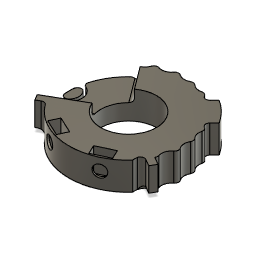
thumbwheelSmall (Autodesk Fusion 360 design; units mm, degrees)
Autodesk Fusion 360 part; units mm, degrees
note: some values were not read from the file. Chosen so that the rebuilt part matches the saved one: which face or edge a step refers to; which pieces of a blend or face edit are solid. Set by a fixed rule: which sketch regions a step uses.
sketch "Sketch1" plane through (0, 0, 0) normal (0, 1, 0) x (1, 0, 0)
  circle A0 centre (0, 0) radius 7
  circle A1 centre (0, 0) radius 15
  line L0 (0, -32.840125) -> (0, 23.247025)
  line L1 (-28.284272, 0) -> (28.284272, 0)
  line L2 (6.339274, 13.594617) -> (-6.339274, -13.594617)
  line L3 (6.339274, 13.594617) -> (-6.339274, -13.594617)
  line L4 (-6.339274, 13.594617) -> (6.339274, -13.594617)
  circle A2 centre (-15, 0) radius 2.5
  circle A3 centre (-15, 0) radius 3.25
  circle A4 centre (0, 16.5) radius 2.5
  circle A5 centre (4.270514, 15.937776) radius 2.5
  circle A6 centre (8.25, 14.289419) radius 2.5
  circle A7 centre (11.667262, 11.667262) radius 2.5
  circle A8 centre (14.289419, 8.25) radius 2.5
  circle A9 centre (15.937776, 4.270514) radius 2.5
  circle A10 centre (16.5, 0) radius 2.5
  circle A11 centre (0, 0) radius 16.5
  circle A12 centre (-4.942275, 15.742424) radius 2.5
  circle A13 centre (15.742424, -4.942275) radius 2.5
  circle A14 centre (-9.430713, 13.539263) radius 2.5
  circle A15 centre (13.539263, -9.430713) radius 2.5
  line L5 (-4.088772, -14.092354) -> (-8.167157, -12.190572)
  line L6 (-8.167157, -12.190572) -> (-7.110612, -9.924802)
  line L7 (-7.110612, -9.924802) -> (-3.032227, -11.826585)
  line L8 (-3.032227, -11.826585) -> (-4.088772, -14.092354)
  line L9 (-4.088772, -14.092354) -> (-7.110612, -9.924802) construction
  line L10 (-8.167157, -12.190572) -> (-3.032227, -11.826585) construction
  line L11 (4.088772, -14.092354) -> (8.167157, -12.190572)
  line L12 (7.110612, -9.924802) -> (3.032227, -11.826585)
  line L13 (4.088772, -14.092354) -> (7.110612, -9.924802) construction
  line L14 (3.032227, -11.826585) -> (4.088772, -14.092354)
  line L15 (8.167157, -12.190572) -> (3.032227, -11.826585) construction
  line L16 (8.167157, -12.190572) -> (7.110612, -9.924802)
  line L17 (0, 0) -> (11.667262, 11.667262)
  line L18 (12.062872, 7.113124) -> (7.113124, 12.062872)
  line L19 (7.113124, 12.062872) -> (11.271652, 16.2214)
  line L20 (11.271652, 16.2214) -> (16.2214, 11.271652)
  line L21 (16.2214, 11.271652) -> (12.062872, 7.113124)
  line L22 (12.062872, 7.113124) -> (11.271652, 16.2214) construction
  line L23 (7.113124, 12.062872) -> (16.2214, 11.271652) construction
  point P0 (-5.599692, -12.008578)
  point P1 (6.339274, -13.594617)
  point P2 (6.339274, -13.594617)
  point P3 (5.599692, -12.008578)
  point P4 (11.667262, 11.667262)
  dimension "d1" = 14
  dimension "d2" = 30
  dimension "d3" = 25
  dimension "d6" = 5
  dimension "d7" = 6.5
  dimension "d8" = 5
  dimension "d10" = -90
  dimension "d36" = 5
  dimension "d37" = 5
  dimension "d38" = 5
  dimension "d39" = 5
  dimension "d47" = 4.5
  dimension "d48" = 2.5
  dimension "d49" = 0.5
  dimension "d60" = 45
  dimension "d61" = 33
  dimension "d62" = 7
  constraint coincident A0.centre A1.centre
  constraint concentric A0 A1
  constraint coincident A0.centre L0
  constraint coincident A0.centre L1
  constraint vertical L0
  constraint horizontal L1
  constraint coincident A0.centre L2
  constraint coincident L1 A2.centre
  constraint coincident A1 A2.centre
  constraint concentric A2 A3
  constraint coincident L0 A4.centre
  constraint concentric A0 A11
  constraint coincident A10.centre A11
  constraint tangent A4 A12
  constraint tangent A12 A14
  constraint tangent A10 A13
  constraint tangent A13 A15
  constraint coincident L3 A0.centre
  constraint perpendicular L5 L6
  constraint parallel L5 L7
  constraint parallel L6 L8
  constraint perpendicular L3 L7
  constraint perpendicular L18 L19
  constraint parallel L18 L20
  constraint parallel L19 L21
  constraint perpendicular L17 L20
  measures "d1" diameter of A0
  measures "d2" diameter of A1
  measures "d3" angle of L0 L2
  measures "d6" diameter of A2
  measures "d7" diameter of A3
  measures "d8" diameter of A4
  measures "d36" diameter of A12
  measures "d37" diameter of A13
  measures "d38" diameter of A14
  measures "d39" diameter of A15
  measures "d60" angle of L1 L17
  measures "d61" diameter of A11
extrude "Extrude1" add sketch "Sketch1" along normal blind 7 contours A0 A1 L1 L4 A10 A13 A15 L11 L12 L16 | A0 A1 L1 A8 A9 A10 L17 L18 | A0 L2 L3 A6 L17 L18 | A0 A1 L0 L4 L11 L12 L14 | A0 A1 L0 L2 L3 A4 A5 A6 | A1 A6 A7 L17 L18 | A1 A7 A8 L17 L18 | A0 A1 L0 L2 L3 L5 L7 L8 | A0 A1 L0 L4 A4 A12 | A0 A1 L1 L4 A3 A14 | A0 A1 L1 L2 L3 A3 L5 L6 L7 | A1 A7 L17 | A1 A7 L17 | A1 A8 L21 | A1 A6 L19 | A1 A6 A7 A11 L17 | A1 A6 A7 | A1 A7 A8 | A1 A7 A8 A11 L17 | A1 A7 A8 A11 L21 | A1 A6 A7 A11 L19 | A1 L1 A2 | A1 L1 A2 | A6 A7 A11 | A7 A8 A11 picked at (7.909113, -7.597993) picked at (9.068114, 6.987484) picked at (7.014257, 9.04726) picked at (1.010742, -11.275528) picked at (1.56298, 11.612023) picked at (8.936312, 10.634324) picked at (10.634324, 8.936312) picked at (-1.010742, -11.275528) picked at (-1.757181, 11.566014) picked at (-10.789506, 3.925439) picked at (-8.435636, -7.427336) picked at (10.608392, 10.139282) picked at (10.139282, 10.608392) picked at (12.382065, 7.951605) picked at (7.951605, 12.382065) picked at (10.248165, 11.960008) picked at (9.148205, 11.912312) picked at (11.912312, 9.148205) picked at (11.960008, 10.248165) picked at (12.961206, 8.95232) picked at (8.95232, 12.961206) picked at (-14.195535, -0.522211) picked at (-14.195535, 0.522211) picked at (9.924324, 12.871109) picked at (12.871109, 9.924324) makes body 1 at (8.102453, 7, -7.979068) makes body 2 at (-12.801016, 2.333333, -1.189314)
sketch "Sketch2" plane through (0, 0, 0) normal (0, -1, 0) x (1, 0, 0)
  arc A0 (8.926881, -13.876628) -> (13.876628, -8.926881) centre (0, 0) ccw
  line L0 (13.876628, -8.926881) -> (12.062872, -7.113124)
  arc A1 (13.836943, -5.791288) -> (12.062872, -7.113124) centre (14.289419, -8.25) ccw
  arc A2 (13.836943, -5.791288) -> (13.879255, -5.689137) centre (0, 0) ccw
  arc A3 (14.864356, -2.01269) -> (13.879255, -5.689137) centre (15.937776, -4.270514) ccw
  arc A4 (14.864356, -2.01269) -> (14.878788, -1.903069) centre (0, 0) ccw
  arc A5 (14.878788, 1.903069) -> (14.878788, -1.903069) centre (16.5, 0) ccw
  arc A6 (14.878788, 1.903069) -> (14.765678, 2.640978) centre (0, 0) ccw
  arc A7 (13.625618, 6.272362) -> (14.765678, 2.640978) centre (15.742424, 4.942275) ccw
  arc A8 (13.625618, 6.272362) -> (13.296674, 6.942511) centre (0, 0) ccw
  arc A9 (11.121244, 10.065681) -> (13.296674, 6.942511) centre (13.539263, 9.430713) ccw
  arc A10 (11.121244, 10.065681) -> (-14.647917, 3.230873) centre (0, 0) ccw
  arc A11 (-14.647917, -3.230873) -> (-14.647917, 3.230873) centre (-15, 0) ccw
  arc A12 (-14.647917, -3.230873) -> (-10.065681, -11.121244) centre (0, 0) ccw
  arc A13 (-6.942511, -13.296674) -> (-10.065681, -11.121244) centre (-9.430713, -13.539263) ccw
  arc A14 (-6.942511, -13.296674) -> (-6.272362, -13.625618) centre (0, 0) ccw
  arc A15 (-2.640978, -14.765678) -> (-6.272362, -13.625618) centre (-4.942275, -15.742424) ccw
  arc A16 (-2.640978, -14.765678) -> (-1.903069, -14.878788) centre (0, 0) ccw
  arc A17 (1.903069, -14.878788) -> (-1.903069, -14.878788) centre (0, -16.5) ccw
  arc A18 (1.903069, -14.878788) -> (2.01269, -14.864356) centre (0, 0) ccw
  arc A19 (5.689137, -13.879255) -> (2.01269, -14.864356) centre (4.270514, -15.937776) ccw
  arc A20 (5.689137, -13.879255) -> (5.791288, -13.836943) centre (0, 0) ccw
  arc A21 (7.113124, -12.062872) -> (5.791288, -13.836943) centre (8.25, -14.289419) ccw
  line L1 (7.113124, -12.062872) -> (8.926881, -13.876628)
  circle A22 centre (0, 0) radius 7
  line L2 (-8.167157, 12.190572) -> (-4.088772, 14.092354)
  line L3 (-4.088772, 14.092354) -> (-3.032227, 11.826585)
  line L4 (-3.032227, 11.826585) -> (-7.110612, 9.924802)
  line L5 (-7.110612, 9.924802) -> (-8.167157, 12.190572)
  line L6 (7.110612, 9.924802) -> (3.032227, 11.826585)
  line L7 (3.032227, 11.826585) -> (4.088772, 14.092354)
  line L8 (4.088772, 14.092354) -> (8.167157, 12.190572)
  line L9 (8.167157, 12.190572) -> (7.110612, 9.924802)
  arc A23 (-14.791667, -2.491304) -> (-14.791667, 2.491304) centre (-15, 0) ccw
  arc A24 (-14.791667, 2.491304) -> (-14.791667, -2.491304) centre (0, 0) ccw
  circle A25 centre (0, 0) radius 15
  constraint concentric A0 A25
extrude "Extrude2" add sketch "Sketch2" against normal blind 1 contours A11 A23 A25 | L2 L3 L4 L5 | L6 L7 L8 L9 picked at (-14.435221, -2.854394) picked at (-4.74387, 11.947914) picked at (4.74387, 11.947914) bodies 1 2
sketch "Sketch3" plane through (0, 7, 0) normal (0, 1, 0) x (-1, 0, 0)
  arc A0 (-5.791288, -13.836943) -> (-5.689137, -13.879255) centre (0, 0) ccw
  arc A1 (-2.01269, -14.864356) -> (-5.689137, -13.879255) centre (-4.270514, -15.937776) ccw
  arc A2 (-2.01269, -14.864356) -> (-1.903069, -14.878788) centre (0, 0) ccw
  arc A3 (1.903069, -14.878788) -> (-1.903069, -14.878788) centre (0, -16.5) ccw
  arc A4 (14.647917, 3.230873) -> (14.647917, -3.230873) centre (15, 0) ccw
  arc A5 (10.065681, -11.121244) -> (14.647917, -3.230873) centre (0, 0) ccw
  circle A6 centre (0, 0) radius 12.5
  line L0 (0, 0) -> (14.647917, -3.230873)
  arc A7 (6.272362, -13.625618) -> (2.640978, -14.765678) centre (4.942275, -15.742424) ccw
  arc A8 (10.065681, -11.121244) -> (6.942511, -13.296674) centre (9.430713, -13.539263) ccw
  line L1 (0, 0) -> (11.979533, 9.027225)
  line L2 (0, 0) -> (0, 15)
  line L3 (0, 0) -> (10.416965, -14.061893)
  line L4 (7.110612, 9.924802) -> (3.032227, 11.826585)
  line L5 (4.088772, 14.092354) -> (8.167157, 12.190572)
  line L6 (8.167157, 12.190572) -> (7.110612, 9.924802)
  arc A9 (-5.791288, -13.836943) -> (-7.113124, -12.062872) centre (-8.25, -14.289419) ccw
  arc A10 (1.903069, -14.878788) -> (2.640978, -14.765678) centre (0, 0) ccw
  arc A11 (-13.876628, -8.926881) -> (-8.926881, -13.876628) centre (0, 0) ccw
  line L7 (-8.926881, -13.876628) -> (-7.113124, -12.062872)
  arc A12 (6.272362, -13.625618) -> (6.942511, -13.296674) centre (0, 0) ccw
  arc A13 (-13.296674, 6.942511) -> (-11.121244, 10.065681) centre (-13.539263, 9.430713) ccw
  arc A14 (-13.296674, 6.942511) -> (-13.625618, 6.272362) centre (0, 0) ccw
  arc A15 (-14.765678, 2.640978) -> (-13.625618, 6.272362) centre (-15.742424, 4.942275) ccw
  arc A16 (-14.765678, 2.640978) -> (-14.878788, 1.903069) centre (0, 0) ccw
  arc A17 (-14.878788, -1.903069) -> (-14.878788, 1.903069) centre (-16.5, 0) ccw
  arc A18 (-14.878788, -1.903069) -> (-14.864356, -2.01269) centre (0, 0) ccw
  arc A19 (-13.879255, -5.689137) -> (-14.864356, -2.01269) centre (-15.937776, -4.270514) ccw
  arc A20 (-13.879255, -5.689137) -> (-13.836943, -5.791288) centre (0, 0) ccw
  arc A21 (-12.062872, -7.113124) -> (-13.836943, -5.791288) centre (-14.289419, -8.25) ccw
  line L8 (-12.062872, -7.113124) -> (-13.876628, -8.926881)
  circle A22 centre (0, 0) radius 7
  line L9 (3.032227, 11.826585) -> (4.088772, 14.092354)
  line L10 (-3.032227, 11.826585) -> (-7.110612, 9.924802)
  line L11 (-7.110612, 9.924802) -> (-8.167157, 12.190572)
  line L12 (-8.167157, 12.190572) -> (-4.088772, 14.092354)
  line L13 (-4.088772, 14.092354) -> (-3.032227, 11.826585)
  circle A23 centre (0, 0) radius 7
  arc A24 (14.647917, 3.230873) -> (-11.121244, 10.065681) centre (0, 0) ccw
  dimension "d46" = 53
  constraint coincident A0.centre A2.centre
  constraint coincident A5 L2.end
  constraint vertical L2
  measures "d46" angle of L1 L2
extrude "Extrude3" cut sketch "Sketch3" 1 faces at (-14.151203, 7, 0) against normal blind 3 contours A4 A5 A6 L0 A8 L3 | A6 L0 L3 A22 A23 | A4 A6 L0 L1 A22 A23 | A4 A6 L0 | A4 A6 L1 A24 picked at (9.960019, -9.910279) picked at (10.246535, -2.869089) picked at (10.246136, 2.09489) picked at (12.593378, -2.372026) picked at (12.900222, 5.788976) on bodies 1 bodies 1
fillet "Fillet1" radius 1 5 edges at (14.878788, 3.5, -1.903069) (14.864356, 3.5, -2.01269) (13.879255, 3.5, -5.689137) (13.836943, 3.5, -5.791288) (14.878788, 3.5, 1.903069) on bodies 1
fillet "Fillet1" radius 1 14 edges at (5.791288, 3.5, -13.836943) (5.689137, 3.5, -13.879255) (2.01269, 3.5, -14.864356) (1.903069, 3.5, -14.878788) (14.765678, 3.5, 2.640978) (-10.065681, 2, -11.121244) (12.062872, 3.5, -7.113124) (7.113124, 3.5, -12.062872) (13.625618, 3.5, 6.272362) (13.296674, 3.5, 6.942511) (-1.903069, 3.5, -14.878788) (-2.640978, 3.5, -14.765678) (-6.272362, 3.5, -13.625618) (-6.942511, 3.5, -13.296674) on bodies 1
sketch "Sketch4" plane through (0, 4, 0) normal (0, 1, 0) x (-1, 0, 0)
  arc A0 (10.439264, -10.77134) -> (14.647917, -3.230873) centre (0, 0) ccw
  line L0 (6.443534, 2.735118) -> (5.590449, 4.212705)
  line L1 (5.590449, 4.212705) -> (14.345029, 9.267165)
  line L2 (14.345029, 9.267165) -> (15.198115, 7.789578)
  line L3 (15.198115, 7.789578) -> (6.443534, 2.735118)
  line L4 (0, -19) -> (0, 26)
  line L5 (-15.198115, 7.789578) -> (-6.443534, 2.735118)
  line L6 (-14.345029, 9.267165) -> (-15.198115, 7.789578)
  line L7 (-5.590449, 4.212705) -> (-14.345029, 9.267165)
  line L8 (-6.443534, 2.735118) -> (-5.590449, 4.212705)
  line L9 (14.771572, 8.528371) -> (0, 0)
  line L10 (0, 0) -> (-14.771572, 8.528371)
  line L11 (11.979533, 9.027225) -> (5.590449, 4.212705)
  arc A1 (14.647917, 3.230873) -> (14.647917, -3.230873) centre (15, 0) ccw
  arc A2 (9.653999, -11.049254) -> (10.439264, -10.77134) centre (9.743313, -10.053251) ccw
  arc A3 (14.647917, 3.230873) -> (11.979533, 9.027225) centre (0, 0) ccw
  arc A4 (4.166786, -5.624757) -> (5.590449, 4.212705) centre (0, 0) ccw
  line L12 (4.166786, -5.624757) -> (8.357241, -11.281464)
  arc A5 (9.653999, -11.049254) -> (8.357241, -11.281464) centre (9.430713, -13.539263) ccw
  point P0 (-17.198214, 3.235958)
  dimension "d44" = 60
  constraint perpendicular L0 L1
  constraint parallel L0 L2
  constraint parallel L1 L3
  constraint vertical L4
  constraint coincident A0.centre L4
  constraint coincident A0.centre L9.end
  constraint perpendicular L0 L9
  measures "d44" angle of L4 L9
extrude "Extrude4" add sketch "Sketch4" along normal blind 3 contours L2 L3 L9 A3 | L3 L9 A3 A4 | L1 L2 L9 A3 | L1 L9 A3 A4 | L1 L11 A3 | L5 L6 L8 L10 | L6 L7 L8 L10 picked at (14.36666, 7.856739) picked at (8.46404, 4.667519) picked at (13.987466, 8.513523) picked at (8.27421, 4.996314) picked at (9.914355, 7.334802) picked at (-11.995559, 6.597287) picked at (-11.569017, 7.33608) bodies 1
extrude "Extrude5" add 2 faces at (-14.129646, 4, 8.267259) (14.177323, 4, 8.000379) along direction (0, -1, 0) blind 3 on bodies 1 bodies 1
fillet "Fillet3" radius 2 1 edges at (-12.990381, 1, 7.5) on bodies 1
fillet "Fillet6" radius 1 8 edges at (11.698439, 4, 7.739155) (-12.542813, 3.5, 8.226655) (-9.919716, 4, 4.742093) (-6.262013, 4, -8.453111) (-14.791667, 2.5, -2.491304) (-14.647917, 2.5, -3.230873) (-14.647917, 2.5, 3.230873) (-14.791667, 2.5, 2.491304) on bodies 1
sketch "Sketch6" plane through (0, 0, 0) normal (0, -1, 0) x (1, 0, 0)
  arc A0 (11.121244, 10.065681) -> (-12.034328, 8.954046) centre (0, 0) ccw
  arc A1 (-12.034328, 8.954046) -> (-13.395898, 6.749067) centre (0, 0) ccw
  arc A2 (11.121244, 10.065681) -> (12.75548, 7.056754) centre (13.539263, 9.430713) ccw
  arc A3 (-13.395898, 6.749067) -> (-10.439264, -10.77134) centre (0, 0) ccw
  arc A4 (-10.439264, -10.77134) -> (-9.653999, -11.049254) centre (-9.743313, -10.053251) ccw
  arc A5 (-7.056754, -12.75548) -> (-9.653999, -11.049254) centre (-9.430713, -13.539263) ccw
  arc A6 (-2.91208, -14.283551) -> (-5.774343, -13.384955) centre (-4.942275, -15.742424) ccw
  arc A7 (1.267961, -14.345406) -> (-1.500002, -14.500001) centre (0, -16.5) ccw
  arc A8 (1.267961, -14.345406) -> (2.488108, -14.184771) centre (1.775145, -13.483569) ccw
  arc A9 (4.937621, -13.528426) -> (2.488108, -14.184771) centre (4.270514, -15.937776) ccw
  arc A10 (4.937621, -13.528426) -> (6.074617, -13.057467) centre (5.204463, -12.564686) ccw
  arc A11 (6.232592, -12.812915) -> (6.074617, -13.057467) centre (8.25, -14.289419) ccw
  arc A12 (7.746662, -12.69641) -> (6.232592, -12.812915) centre (7.039555, -13.403516) ccw
  line L0 (7.746662, -12.69641) -> (8.926881, -13.876628)
  arc A13 (8.926881, -13.876628) -> (13.876628, -8.926881) centre (0, 0) ccw
  line L1 (13.876628, -8.926881) -> (12.69641, -7.746662)
  arc A14 (12.812915, -6.232592) -> (12.69641, -7.746662) centre (13.403516, -7.039555) ccw
  arc A15 (13.057467, -6.074617) -> (12.812915, -6.232592) centre (14.289419, -8.25) ccw
  arc A16 (13.057467, -6.074617) -> (13.528426, -4.937621) centre (12.564686, -5.204463) ccw
  arc A17 (14.184771, -2.488108) -> (13.528426, -4.937621) centre (15.937776, -4.270514) ccw
  arc A18 (14.184771, -2.488108) -> (14.345406, -1.267961) centre (13.483569, -1.775145) ccw
  arc A19 (14.500001, 1.500002) -> (14.345406, -1.267961) centre (16.5, 0) ccw
  arc A20 (14.500001, 1.500002) -> (14.283551, 2.91208) centre (13.700002, 2.100003) ccw
  arc A21 (13.384955, 5.774343) -> (14.283551, 2.91208) centre (15.742424, 4.942275) ccw
  arc A22 (13.384955, 5.774343) -> (12.75548, 7.056754) centre (12.441967, 6.10717) ccw
  circle A23 centre (0, 0) radius 7
  arc A24 (-7.056754, -12.75548) -> (-5.774343, -13.384955) centre (-6.10717, -12.441967) ccw
  arc A25 (-2.91208, -14.283551) -> (-1.500002, -14.500001) centre (-2.100003, -13.700002) ccw
sketch "Sketch7" plane through (-5.071419, 0, 10.875693) normal (-0.422618, 0, 0.906308) x (0.906308, 0, 0.422618)
  line L0 (2.25, 1) -> (2.25, 7)
  line L1 (2.25, 7) -> (-2.25, 7)
  circle A0 centre (0, 4) radius 1.5
  line L2 (-2.25, 7) -> (-2.25, 1)
  line L3 (-2.25, 1) -> (2.25, 1)
  point P0 (0, 7)
  point P1 (2.25, 4)
  dimension "d52" = 3
  constraint midpoint L1 P0
  constraint midpoint L0 P1
  constraint vertical A0.centre P0
  constraint horizontal A0.centre P1
  measures "d52" diameter of A0
extrude "Extrude8" cut sketch "Sketch7" along normal blind 5 contours A0 picked at (-0.133474, 4.340086) bodies 1
sketch "Sketch8" plane through (5.071419, 0, 10.875693) normal (0.422618, 0, 0.906308) x (0.906308, 0, -0.422618)
  line L0 (2.25, 1) -> (2.25, 7)
  line L1 (2.25, 7) -> (-2.25, 7)
  line L2 (-2.25, 7) -> (-2.25, 1)
  circle A0 centre (0, 4) radius 1.5
  line L3 (-2.25, 1) -> (2.25, 1)
  point P0 (0, 7)
  point P1 (2.25, 4)
  dimension "d55" = 3
  constraint midpoint L1 P0
  constraint midpoint L0 P1
  constraint horizontal A0.centre P1
  constraint vertical A0.centre P0
  measures "d55" diameter of A0
extrude "Extrude9" cut sketch "Sketch8" along normal blind 5 contours A0 picked at (0.383155, 4.412943) bodies 1
fillet "Fillet9" radius 1 2 edges at (13.041995, 1, 6.907149) (11.682157, 1, 7.757048) on bodies 1
